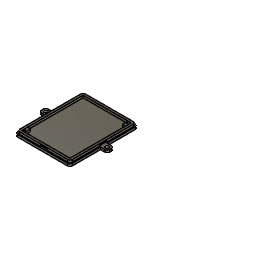
Enclosure-Rear-Cover (Autodesk Fusion 360 design; units mm, degrees)
Autodesk Fusion 360 part; units mm, degrees
sketch "Sketch1" plane through (0, 0, -4.069) normal (0, 0, -1) x (-1, 0, 0)
  line L0 (-14.51, 64.76) -> (-14.51, 40.46)
  line L1 (-14.76, 40.46) -> (-14.76, 34.46)
  line L2 (-61.36, 10.16) -> (-61.36, 34.46)
  line L3 (-61.11, 34.46) -> (-61.11, 40.46)
  line L4 (-62.36, 65.76) -> (-62.36, 9.16)
  line L5 (-13.51, 9.16) -> (-13.51, 65.76)
  arc A0 (-60.86, 10.66) -> (-58.86, 8.66) centre (-58.86, 10.66) ccw
  line L6 (-17.01, 8.66) -> (-58.86, 8.66)
  line L7 (-59.36, 64.76) -> (-16.51, 64.76)
  line L8 (-54.0908, 10.16) -> (-43.1668, 10.16)
  line L9 (-58.86, 66.26) -> (-17.01, 66.26)
  line L10 (-42.45, 9.0382) -> (-33.83, 9.0382)
  line L11 (-54.0908, 10.16) -> (-54.0908, 9.0382)
  line L12 (-59.36, 64.76) -> (-16.51, 64.76)
  line L13 (-54.0908, 10.16) -> (-59.36, 10.16)
  line L14 (-22.1792, 9.0382) -> (-54.0908, 9.0382)
  line L15 (-34.5959, 10.16) -> (-22.1792, 10.16)
  line L16 (-16.51, 66.76) -> (-59.36, 66.76)
  line L17 (-58.86, 8.66) -> (-17.01, 8.66)
  line L18 (-43.1668, 10.16) -> (-34.5959, 10.16)
  arc A1 (-60.86, 10.66) -> (-58.86, 8.66) centre (-58.86, 10.66) ccw
  line L19 (-17.01, 8.66) -> (-58.86, 8.66)
  line L20 (-17.01, 66.26) -> (-58.86, 66.26)
  arc A2 (-61.36, 10.16) -> (-59.36, 8.16) centre (-59.36, 10.16) ccw
  arc A3 (-61.36, 10.16) -> (-59.36, 8.16) centre (-59.36, 10.16) ccw
  line L21 (-54.0908, 9.0382) -> (-22.1792, 9.0382)
  line L22 (-58.86, 66.26) -> (-17.01, 66.26)
  line L23 (-59.36, 8.16) -> (-16.51, 8.16)
  arc A4 (-60.86, 10.66) -> (-58.86, 8.66) centre (-58.86, 10.66) ccw
  line L24 (-16.51, 66.76) -> (-59.36, 66.76)
  line L25 (-15.01, 64.26) -> (-15.01, 10.66)
  line L26 (-16.51, 64.76) -> (-16.51, 10.16)
  line L27 (-15.51, 34.46) -> (-15.01, 34.46)
  line L28 (-15.01, 34.46) -> (-15.01, 10.66)
  line L29 (-7.51, 40.46) -> (-7.51, 34.46)
  line L30 (-14.51, 10.16) -> (-14.51, 64.76)
  line L31 (-15.01, 10.66) -> (-15.01, 64.26)
  line L32 (-60.86, 10.66) -> (-60.86, 64.26)
  line L33 (-61.36, 64.76) -> (-61.36, 10.16)
  line L34 (-60.86, 64.26) -> (-60.86, 10.66)
  line L35 (-59.36, 10.16) -> (-59.36, 64.76)
  line L36 (-61.36, 64.76) -> (-61.36, 10.16)
  line L37 (-16.51, 64.76) -> (-16.51, 10.16)
  line L38 (-14.51, 10.16) -> (-14.51, 64.76)
  line L39 (-60.86, 10.66) -> (-60.86, 34.46)
  line L40 (-15.01, 64.26) -> (-15.01, 40.46)
  line L41 (-15.01, 40.46) -> (-15.51, 40.46)
  line L42 (-15.51, 40.46) -> (-15.51, 34.46)
  line L43 (-16.51, 10.16) -> (-22.1792, 10.16)
  line L44 (-59.36, 10.16) -> (-59.36, 64.76)
  line L45 (-15.01, 40.46) -> (-7.51, 40.46)
  line L46 (-22.1792, 10.16) -> (-22.1792, 9.0382)
  line L47 (-15.01, 34.46) -> (-15.01, 40.46)
  arc A5 (-17.01, 8.66) -> (-15.01, 10.66) centre (-17.01, 10.66) ccw
  arc A6 (-15.01, 64.26) -> (-17.01, 66.26) centre (-17.01, 64.26) ccw
  circle A7 centre (-10.51, 37.46) radius 1.5
  arc A8 (-58.86, 66.26) -> (-60.86, 64.26) centre (-58.86, 64.26) ccw
  arc A9 (-59.36, 66.76) -> (-61.36, 64.76) centre (-59.36, 64.76) ccw
  line L48 (-60.86, 40.46) -> (-68.36, 40.46)
  line L49 (-68.36, 40.46) -> (-68.36, 34.46)
  line L50 (-68.36, 34.46) -> (-60.86, 34.46)
  line L51 (-60.86, 34.46) -> (-60.86, 40.46)
  arc A10 (-14.51, 64.76) -> (-16.51, 66.76) centre (-16.51, 64.76) ccw
  arc A11 (-58.86, 66.26) -> (-60.86, 64.26) centre (-58.86, 64.26) ccw
  arc A12 (-58.86, 66.26) -> (-60.86, 64.26) centre (-58.86, 64.26) ccw
  circle A13 centre (-65.36, 37.46) radius 1.5
  line L52 (-60.86, 40.46) -> (-60.86, 64.26)
  line L53 (-16.51, 10.16) -> (-59.36, 10.16)
  line L54 (-59.36, 8.16) -> (-16.51, 8.16)
  line L55 (-60.36, 34.46) -> (-60.36, 40.46)
  arc A14 (-16.51, 8.16) -> (-14.51, 10.16) centre (-16.51, 10.16) ccw
  line L56 (-54.0908, 9.0382) -> (-54.0908, 10.16)
  line L57 (-60.86, 34.46) -> (-60.36, 34.46)
  arc A15 (-15.01, 64.26) -> (-17.01, 66.26) centre (-17.01, 64.26) ccw
  line L58 (-60.36, 40.46) -> (-60.86, 40.46)
  arc A16 (-15.01, 64.26) -> (-17.01, 66.26) centre (-17.01, 64.26) ccw
  arc A17 (-17.01, 8.66) -> (-15.01, 10.66) centre (-17.01, 10.66) ccw
  arc A18 (-59.36, 66.76) -> (-61.36, 64.76) centre (-59.36, 64.76) ccw
  line L59 (-7.51, 34.46) -> (-15.01, 34.46)
  arc A19 (-17.01, 8.66) -> (-15.01, 10.66) centre (-17.01, 10.66) ccw
  arc A20 (-16.51, 8.16) -> (-14.51, 10.16) centre (-16.51, 10.16) ccw
  arc A21 (-14.51, 64.76) -> (-16.51, 66.76) centre (-16.51, 64.76) ccw
  arc A22 (-60.36, 67.76) -> (-62.36, 65.76) centre (-60.36, 65.76) ccw
  arc A23 (-62.36, 9.16) -> (-60.36, 7.16) centre (-60.36, 9.16) ccw
  arc A24 (-15.51, 7.16) -> (-13.51, 9.16) centre (-15.51, 9.16) ccw
  arc A25 (-13.51, 65.76) -> (-15.51, 67.76) centre (-15.51, 65.76) ccw
  line L60 (-16.51, 8.16) -> (-59.36, 8.16)
  line L61 (-59.36, 66.76) -> (-16.51, 66.76)
  line L62 (-60.36, 7.16) -> (-15.51, 7.16)
  line L63 (-15.51, 67.76) -> (-60.36, 67.76)
  arc A26 (-14.51, 64.76) -> (-16.51, 66.76) centre (-16.51, 64.76) ccw
  arc A27 (-16.51, 8.16) -> (-14.51, 10.16) centre (-16.51, 10.16) ccw
  arc A28 (-61.36, 10.16) -> (-59.36, 8.16) centre (-59.36, 10.16) ccw
  arc A29 (-59.36, 66.76) -> (-61.36, 64.76) centre (-59.36, 64.76) ccw
  arc A30 (-60.36, 67.76) -> (-62.36, 65.76) centre (-60.36, 65.76) ccw
  arc A31 (-13.51, 65.76) -> (-15.51, 67.76) centre (-15.51, 65.76) ccw
  arc A32 (-13.51, 65.76) -> (-15.51, 67.76) centre (-15.51, 65.76) ccw
  arc A33 (-15.51, 7.16) -> (-13.51, 9.16) centre (-15.51, 9.16) ccw
  arc A34 (-62.36, 9.16) -> (-60.36, 7.16) centre (-60.36, 9.16) ccw
  line L64 (-60.36, 7.16) -> (-15.51, 7.16)
  line L65 (-13.51, 9.16) -> (-13.51, 65.76)
  line L66 (-15.51, 67.76) -> (-60.36, 67.76)
  line L67 (-62.36, 65.76) -> (-62.36, 9.16)
  line L68 (-14.51, 40.46) -> (-14.76, 40.46)
  line L69 (-14.76, 34.46) -> (-14.51, 34.46)
  line L70 (-14.51, 34.46) -> (-14.51, 10.16)
  line L71 (-61.36, 34.46) -> (-61.11, 34.46)
  line L72 (-61.11, 40.46) -> (-61.36, 40.46)
  line L73 (-61.36, 40.46) -> (-61.36, 64.76)
  point P0 (-10.51, 37.46)
  point P1 (-65.36, 37.46)
  dimension "d210" = 6
  dimension "d211" = 7.5
  dimension "d212" = 7.5
  dimension "d213" = 6
  dimension "d214" = 3
  dimension "d215" = 3
  dimension "d216" = 3
  dimension "d217" = 3
  dimension "d218" = 3
  dimension "d219" = 3
  constraint coincident L9.start L20.end
  constraint coincident L9.end L20.start
  constraint coincident L25.start L31.end
  constraint coincident L25.end L28.end
  constraint coincident L6.start L17.end
  constraint coincident A0.end L6.end
  constraint coincident A0.start A1.start
  constraint coincident L32.end L34.start
  constraint coincident A2.end A3.end
  constraint coincident L23.end L54.end
  constraint coincident L30.start L38.start
  constraint coincident L0.start L30.end
  constraint coincident L16.start L24.start
  constraint coincident L16.end L24.end
  constraint coincident L33.start L36.start
  constraint coincident L2.start A2.start
  constraint horizontal L12
  constraint vertical L26
  constraint horizontal L53
  constraint vertical L44
  constraint coincident L26.end L37.end
  constraint coincident L7.start L12.start
  constraint horizontal L48
  constraint vertical L49
  constraint horizontal L50
  constraint vertical L51
  constraint coincident L48.start L51.end
  constraint horizontal L45
  constraint vertical L29
  constraint horizontal L59
  constraint vertical L47
  constraint coincident L40.end L41.start
  constraint coincident P1 A13.centre
  constraint coincident P0 A7.centre
  constraint coincident A22.start L63.end
  constraint coincident L4.start A22.end
  constraint coincident L5.end A25.start
  constraint coincident A25.end L63.start
  constraint tangent L5 A32
  constraint tangent L5 A33
  constraint coincident A24.start L62.end
  constraint coincident L5.start A24.end
  constraint tangent L4 A34
  constraint tangent L62 A34
  constraint coincident L4.end A23.start
  constraint tangent A33 L64
  constraint tangent A30 L66
  measures "d210" distance of L48.start L39.end
  measures "d211" distance of L48.start L48.end
  measures "d212" distance of L40.end L29.start
  measures "d213" distance of L27.end L40.end
  measures "d214" distance of P1 L49
  measures "d215" distance of P1 L48
  measures "d216" distance of P0 L29
  measures "d217" distance of P0 L59
  measures "d218" diameter of A13
  measures "d219" diameter of A7
extrude "Extrude1" add sketch "Sketch1" along normal blind 2 contours L0 L4 L5 L16 L24 L30 L33 L36 L38 L45 A9 L48 A10 A18 A21 A22 A25 L61 L63 A26 A29 A30 A31 A32 L65 L66 L67 L73 | L0 L9 L16 L20 L22 L24 L25 L30 L31 L32 L33 L34 L36 L38 L40 L45 A6 A8 A9 L48 A10 A11 A12 L52 A15 A16 A18 A21 L61 A26 A29 L68 L72 L73 | L5 L30 L38 L45 L59 L65 | L1 L30 L38 L45 L59 L68 L69 | L2 L4 L5 A2 A3 L23 L30 L33 L36 L38 L50 L54 A14 L59 A20 A23 A24 L60 L62 A27 A28 A33 A34 L64 L65 L67 L70 | L2 A0 L6 L17 A1 L19 A2 A3 L23 A4 L25 L28 L30 L31 L32 L33 L34 L36 L38 L39 A5 L50 L54 A14 A17 L59 A19 A20 L60 A27 A28 L69 L70 L71 | L1 L25 L31 L45 L47 L59 | L5 L29 L45 L59 L65 | A0 L6 L9 L17 A1 L19 L20 L22 A4 L25 L27 L28 L31 L32 L34 L39 L40 L41 L42 A5 A6 A8 A11 A12 L52 L55 L57 A15 L58 A16 A17 A19 | L25 L27 L31 L41 L42 L47 | L3 L33 L36 L48 L50 L71 L72 | L4 L33 L36 L48 L50 L67 | L3 L32 L34 L48 L50 L51 | L4 L48 L49 L50 L67 | L32 L34 L51 L55 L57 L58 | L7 L8 L12 L13 L15 L18 L26 L35 L37 L43 L44 L53 | L8 L10 L11 L14 L15 L18 L21 L46 L53 L56 makes body 1
extrude "Extrude2" add sketch "Sketch1" against normal blind 2 contours L0 L9 L16 L20 L22 L24 L25 L30 L31 L32 L33 L34 L36 L38 L40 L45 A6 A8 A9 L48 A10 A11 A12 L52 A15 A16 A18 A21 L61 A26 A29 L68 L72 L73 | L1 L30 L38 L45 L59 L68 L69 | L2 A0 L6 L17 A1 L19 A2 A3 L23 A4 L25 L28 L30 L31 L32 L33 L34 L36 L38 L39 A5 L50 L54 A14 A17 L59 A19 A20 L60 A27 A28 L69 L70 L71 | L1 L25 L31 L45 L47 L59 | A0 L6 L9 L17 A1 L19 L20 L22 A4 L25 L27 L28 L31 L32 L34 L39 L40 L41 L42 A5 A6 A8 A11 A12 L52 L55 L57 A15 L58 A16 A17 A19 | L25 L27 L31 L41 L42 L47 | L3 L33 L36 L48 L50 L71 L72 | L3 L32 L34 L48 L50 L51 | L32 L34 L51 L55 L57 L58 | L8 L10 L11 L14 L15 L18 L21 L46 L53 L56 bodies 1
sketch "Sketch2" plane through (14.51, 0, 0) normal (-1, 0, 0) x (0, 0, 1)
  line L0 (-2.069, 64.26, -0.5) -> (-4.069, 64.26, -0.5)
  line L1 (-4.069, 10.66, -0.5) -> (-2.069, 10.66, -0.5)
  line L2 (-4.069, 10.66, -0.5) -> (-4.069, 64.26, -0.5)
  line L3 (-2.069, 10.66, -0.5) -> (-2.069, 64.26, -0.5)
  line L4 (-4.069, 40.46, -0.5) -> (-4.069, 34.46, -0.5)
  line L5 (-2.069, 64.26, -0.5) -> (-2.069, 10.66, -0.5)
  line L6 (-3.069, 34.46, -0.5) -> (-3.069, 40.46, -0.5)
  line L7 (-4.069, 64.26, -0.5) -> (-4.069, 10.66, -0.5)
  line L8 (-4.069, 64.26, -0.5) -> (-2.069, 64.26, -0.5)
  line L9 (-2.069, 10.66, -0.5) -> (-4.069, 10.66, -0.5)
  line L10 (-3.069, 40.46, -0.5) -> (-4.069, 40.46, -0.5)
  line L11 (-4.069, 34.46, -0.5) -> (-3.069, 34.46, -0.5)
  line L12 (-4.069, 64.26, -0.5) -> (-4.069, 10.66, -0.5)
  line L13 (-2.069, 10.16) -> (-2.069, 64.76)
  line L14 (-2.069, 64.76) -> (-4.069, 64.76)
  line L15 (-4.069, 64.76) -> (-4.069, 10.16)
  line L16 (-4.069, 10.16) -> (-2.069, 10.16)
  line L17 (-3.0991, 40.46, -0.5) -> (-4.069, 40.46, 0)
  line L18 (-4.069, 40.46) -> (-4.069, 34.4301)
  line L19 (-4.069, 34.4301) -> (-3.0991, 34.4301)
  line L20 (-3.0991, 34.4301, 0) -> (-3.0991, 40.46, -0.5)
  line L21 (-3, 40.5) -> (-4.069, 40.5)
  line L22 (-4.069, 40.5) -> (-4.069, 34.4301)
  line L23 (-4.069, 34.4301) -> (-3, 34.4301)
  line L24 (-3, 34.4301) -> (-3, 40.5)
  dimension "d224" = 6
  dimension "d225" = 23.8
  dimension "d226" = 1
  constraint vertical L18
  constraint horizontal L19
  constraint coincident L15 L18.end
  constraint horizontal L21
  constraint vertical L22
  constraint horizontal L23
  constraint vertical L24
extrude "Extrude3" cut sketch "Sketch2" against normal blind 0.5 contours L15 L18 L19 L21 L22 L23 L24 bodies 1
sketch "Sketch3" plane through (61.36, 0, 0) normal (1, 0, 0) x (0, 0, -1)
  line L0 (4.069, 10.16) -> (4.069, 64.76)
  line L1 (3.069, 34.46) -> (4.069, 34.46)
  line L2 (4.069, 34.46) -> (4.069, 40.46)
  line L3 (4.069, 40.46) -> (3.069, 40.46)
  line L4 (3.069, 40.46) -> (3.069, 34.46)
  line L5 (4.069, 64.76) -> (2.069, 64.76)
  line L6 (2.069, 64.76) -> (2.069, 10.16)
  line L7 (2.069, 10.16) -> (4.069, 10.16)
  constraint horizontal L1
  constraint vertical L2
  constraint horizontal L3
  constraint vertical L4
  constraint coincident L0 L2.end
extrude "Extrude4" cut sketch "Sketch3" against normal blind 0.5 contours L0 L1 L2 L3 L4 bodies 1
chamfer "Chamfer1" distance 0.5 distance2 0.5 2 edges at (61.36, 37.46, -3.069) (14.51, 37.465, -3) measured on face at (61.36, 56.66, -3.069) measured on face at (14.51, 18.25, -3.046) on bodies 1
fillet "Fillet1" radius 2 4 edges at (68.36, 40.46, -5.069) (68.36, 34.46, -5.069) (7.51, 40.46, -5.069) (7.51, 34.46, -5.069) on bodies 1
sketch "Sketch4" plane through (0, 0, -4.069) normal (0, 0, 1) x (1, 0, 0)
  line L0 (16.51, 10.16) -> (59.36, 10.16)
  line L1 (59.36, 10.16) -> (59.36, 64.76)
  line L2 (59.36, 64.76) -> (16.51, 64.76)
  line L3 (16.51, 64.76) -> (16.51, 10.16)
  line L4 (59.36, 64.76) -> (56.66, 64.76)
  line L5 (56.66, 64.76) -> (56.66, 59.76)
  line L6 (56.66, 59.76) -> (59.36, 59.76)
  line L7 (59.36, 59.76) -> (59.36, 64.76)
  line L8 (16.51, 10.16) -> (19.21, 10.16)
  line L9 (19.21, 10.16) -> (19.21, 15.16)
  line L10 (19.21, 15.16) -> (16.51, 15.16)
  line L11 (16.51, 15.16) -> (16.51, 10.16)
  dimension "d263" = 2.7
  dimension "d264" = 5
  dimension "d265" = 2.7
  dimension "d266" = 5
  constraint horizontal L4
  constraint vertical L5
  constraint horizontal L6
  constraint vertical L7
  constraint coincident L1.end L2.start
  constraint horizontal L8
  constraint vertical L9
  constraint horizontal L10
  constraint vertical L11
  constraint coincident L0.start L3.end
  measures "d263" distance of L1.end L4.end
  measures "d264" distance of L1.end L6.end
  measures "d265" distance of L0.start L8.end
  measures "d266" distance of L0.start L10.end
extrude "Extrude5" add sketch "Sketch4" along normal blind 2 separate body contours L0 L3 L8 L9 L10 L11 | L1 L2 L4 L5 L6 L7 makes body 2 at (58.46, 61.4267, -4.069) makes body 3 at (17.41, 13.4933, -4.069)
sketch "Sketch5" plane through (0, 0, -6.069) normal (0, 0, -1) x (-1, 0, 0)
  arc A0 (-9.51, 34.46) -> (-7.51, 36.46) centre (-9.51, 36.46) ccw
  line L0 (-7.51, 36.46) -> (-7.51, 38.46)
  arc A1 (-7.51, 38.46) -> (-9.51, 40.46) centre (-9.51, 38.46) ccw
  line L1 (-9.51, 40.46) -> (-13.51, 40.46)
  line L2 (-13.51, 40.46) -> (-13.51, 65.76)
  arc A2 (-13.51, 65.76) -> (-15.51, 67.76) centre (-15.51, 65.76) ccw
  line L3 (-15.51, 67.76) -> (-60.36, 67.76)
  arc A3 (-60.36, 67.76) -> (-62.36, 65.76) centre (-60.36, 65.76) ccw
  line L4 (-62.36, 65.76) -> (-62.36, 40.46)
  line L5 (-62.36, 40.46) -> (-66.36, 40.46)
  arc A4 (-66.36, 40.46) -> (-68.36, 38.46) centre (-66.36, 38.46) ccw
  line L6 (-68.36, 38.46) -> (-68.36, 36.46)
  arc A5 (-68.36, 36.46) -> (-66.36, 34.46) centre (-66.36, 36.46) ccw
  line L7 (-66.36, 34.46) -> (-62.36, 34.46)
  line L8 (-62.36, 34.46) -> (-62.36, 9.16)
  arc A6 (-62.36, 9.16) -> (-60.36, 7.16) centre (-60.36, 9.16) ccw
  line L9 (-60.36, 7.16) -> (-15.51, 7.16)
  arc A7 (-15.51, 7.16) -> (-13.51, 9.16) centre (-15.51, 9.16) ccw
  line L10 (-13.51, 9.16) -> (-13.51, 34.46)
  line L11 (-13.51, 34.46) -> (-9.51, 34.46)
  circle A8 centre (-65.36, 37.46) radius 1.5
  circle A9 centre (-10.51, 37.46) radius 1.5
  circle A10 centre (-57.785, 62.865) radius 0.75
  circle A11 centre (-17.78, 11.43) radius 0.75
  circle A12 centre (-57.785, 62.865) radius 0.75
  circle A13 centre (-17.78, 11.43) radius 0.75
  constraint concentric A10 A12
  constraint concentric A11 A13
hole "Hole1" at (17.78, 11.43, -6.069) at (57.785, 62.865, -6.069) direction (0, 0, 1) diameter 0.9 end up to surface (4 mm away) countersink diameter 2 countersink angle 90 bodies 1 2 3
sketch "Sketch6" plane through (0, 8.16, 0) normal (0, -1, 0) x (1, 0, 0)
  line L0 (16.51, -4.069) -> (59.36, -4.069)
  line L1 (59.36, -4.069) -> (59.36, -2.069)
  line L2 (59.36, -2.069) -> (16.51, -2.069)
  line L3 (16.51, -2.069) -> (16.51, -4.069)
  line L4 (34.935, -4.069) -> (40.935, -4.069)
  line L5 (40.935, -4.069) -> (40.935, -3.069)
  line L6 (40.935, -3.069) -> (34.935, -3.069)
  line L7 (34.935, -3.069) -> (34.935, -4.069)
  dimension "d307" = 6
  dimension "d308" = 1
  dimension "d309" = 42.85
  dimension "d310" = 18.425
  constraint horizontal L4
  constraint vertical L5
  constraint horizontal L6
  constraint vertical L7
  constraint coincident L0 L4.start
  measures "d307" distance of L4.start L4.end
  measures "d308" distance of L4.start L6.end
  measures "d309" distance of L1.end L2.end
  measures "d310" distance of L3 L7
extrude "Extrude6" cut sketch "Sketch6" against normal blind 0.5 contours L0 L4 L5 L6 L7 bodies 1
sketch "Sketch7" plane through (0, 66.76, 0) normal (0, 1, 0) x (-1, 0, 0)
  line L0 (-59.36, -4.069) -> (-16.51, -4.069)
  line L1 (-16.51, -4.069) -> (-16.51, -2.069)
  line L2 (-16.51, -2.069) -> (-59.36, -2.069)
  line L3 (-59.36, -2.069) -> (-59.36, -4.069)
  line L4 (-34.935, -3.069) -> (-34.935, -4.069)
  line L5 (-34.935, -4.069) -> (-40.935, -4.069)
  line L6 (-40.935, -4.069) -> (-40.935, -3.069)
  line L7 (-40.935, -3.069) -> (-34.935, -3.069)
  line L8 (-40.935, -3.069) -> (-34.935, -3.069)
  line L9 (-34.935, -3.069) -> (-34.935, -4.069)
  line L10 (-34.935, -4.069) -> (-40.935, -4.069)
  line L11 (-40.935, -4.069) -> (-40.935, -3.069)
  constraint horizontal L8
  constraint vertical L9
  constraint horizontal L10
  constraint vertical L11
  constraint coincident L4.end L5.start
  constraint coincident L6.end L7.start
extrude "Extrude7" cut sketch "Sketch7" against normal blind 0.5 contours L0 L4 L5 L6 L7 L8 L9 L10 L11 bodies 1
chamfer "Chamfer2" distance 0.5 angle 45 2 edges at (37.935, 66.76, -3.069) (37.935, 8.16, -3.069) on bodies 1
equation "d222 = StackLipHeight"
equation "d224 = NotchLength"
equation "d225 = NotchOffset"
equation "d226 = NotchWidth"
equation "d229 = NotchDepth"
equation "d263 = BoardSupportWidth"
equation "d264 = BoardSupportLong"
equation "d265 = BoardSupportWidth"
equation "d266 = BoardSupportLong"
equation "d307 = NotchLength"
equation "d308 = NotchWidth"
equation "d310 = ( 42.85 mm - NotchLength ) / 2"
equation "BoardSupportWidth = 2.7 mm"
equation "BoardSupportLong = 5 mm"
equation "StackLipHeight = -2 mm"
equation "d168 = NotchLength"
equation "NotchDepth = -0.5 mm"
equation "NotchLength = 6 mm"
equation "NotchOffset = ( d285 - d168 ) / 2"
equation "NotchWidth = 1.00 mm"
equation "d285 = 53.60 mm"
